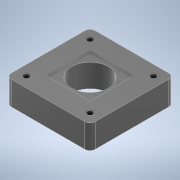
# Autodesk Inventor part: Base
Saved by Autodesk Inventor 2022 (Build 260153000, 153)
## iProperties
Created: 2022-03-02
Part Number: Base
Material: Genérico
Document SubType Name: Modeling
Designer: JK
Density: 1 g/cm^3
Appearance: Suave - Negro
Author: JK
Autodesk Inventor part; units mm, degrees
ref_plane "YZ Plane" through (0, 0, 0) normal (1, 0, 0) x (0, 1, 0)
ref_plane "XZ Plane" through (0, 0, 0) normal (0, 1, 0) x (-1, 0, 0)
ref_plane "XY Plane" through (0, 0, 0) normal (0, 0, 1) x (1, 0, 0)
sketch "Boceto1" plane through (0, 0, 0) normal (0, 1, 0) x (-1, 0, 0)
  line L0 (-41.2, 41.2) -> (41.2, 41.2)
  line L1 (41.2, 41.2) -> (41.2, -41.2)
  line L2 (41.2, -41.2) -> (-41.2, -41.2)
  line L3 (-41.2, -41.2) -> (-41.2, 41.2)
  line L4 (-41.2, 41.2) -> (41.2, -41.2) construction
  line L5 (41.2, 41.2) -> (-41.2, -41.2) construction
  circle A0 centre (0, 0) radius 18.2
  dimension "d0" = 82.4
  dimension "d1" = 82.4
  dimension "d2" = 36.4
  constraints: 12 end point, 2 midpoint, 2 parallel, 1 centre point, 1 coincident, 1 horizontal, 1 perpendicular
  measures "d0" distance of L0.end L1.end
  measures "d1" distance of L1.end L2.end
  measures "d2" diameter of A0
extrude "Extrusión1" add sketch "Boceto1" along normal blind 22.5
sketch "Boceto2" plane through (0, 22.5, 0) normal (0, 1, 0) x (1, 0, 0)
  circle A0 centre (-31.2, -31.2) radius 2.7
  line L0 (-41.2, 41.2) -> (-41.2, -41.2) projected
  line L1 (-41.2, -41.2) -> (41.2, -41.2) projected
  point P0 (0, 0)
  dimension "d5" = 5.4
  dimension "d6" = 10
  dimension "d7" = 10
  constraints: 1 centre point
  measures "d5" diameter of A0
  measures "d6" distance from line of L0 A0.centre
  measures "d7" distance from line of L1 A0.centre
extrude "Extrusión2" cut sketch "Boceto2" against normal through all
pattern_circular "Patrón circular1" count 4 over 360 about axis through (0, 0, 0) along (0, 1, 0) of "Extrusión2"
fillet "Empalme1" radius 5 4 edges at (-41.2, 11.25, 41.2) (41.2, 11.25, 41.2) (41.2, 11.25, -41.2) (-41.2, 11.25, -41.2)
sketch "Boceto3" plane through (0, 22.5, 0) normal (0, 1, 0) x (1, 0, 0)
  line L0 (-21.2, -21.2) -> (21.2, -21.2)
  line L1 (21.2, -21.2) -> (21.2, 21.2)
  line L2 (21.2, 21.2) -> (-21.2, 21.2)
  line L3 (-21.2, 21.2) -> (-21.2, -21.2)
  line L4 (-21.2, -21.2) -> (21.2, 21.2) construction
  line L5 (21.2, -21.2) -> (-21.2, 21.2) construction
  arc A0 (-36.2, 41.2) -> (-41.2, 36.2) centre (-36.2, 36.2) ccw projected
  line L6 (-41.2, 36.2) -> (-41.2, -36.2) projected
  arc A1 (-41.2, -36.2) -> (-36.2, -41.2) centre (-36.2, -36.2) ccw projected
  line L7 (-36.2, -41.2) -> (36.2, -41.2) projected
  arc A2 (36.2, -41.2) -> (41.2, -36.2) centre (36.2, -36.2) ccw projected
  line L8 (41.2, -36.2) -> (41.2, 36.2) projected
  arc A3 (41.2, 36.2) -> (36.2, 41.2) centre (36.2, 36.2) ccw projected
  line L9 (36.2, 41.2) -> (-36.2, 41.2) projected
  circle A4 centre (-31.2, 31.2) radius 2.7 projected
  circle A5 centre (31.2, 31.2) radius 2.7 projected
  circle A6 centre (31.2, -31.2) radius 2.7 projected
  circle A7 centre (-31.2, -31.2) radius 2.7 projected
  circle A8 centre (0, 0) radius 18.2 projected
  dimension "d14" = 42.4
  dimension "d15" = 42.4
  constraints: 12 end point, 2 midpoint, 2 parallel, 1 horizontal, 1 perpendicular
  measures "d14" distance of L1.end L2.end
  measures "d15" distance of L0.end L1.end
extrude "Extrusión3" add sketch "Boceto3" along normal blind 1 contours L9 A3 L8 A2 L7 A1 L6 A0
